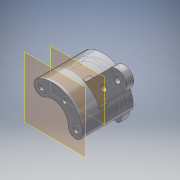
# Autodesk Inventor part: ChasssiPrototypeA2
Saved by Autodesk Inventor 2017 (Build 210142000, 142)
## iProperties
Created: 2018-04-20
Part Number: ChasssiPrototypeA2
Material: PC/ABS Plastic
Document SubType Name: Modeling
Designer: MtgSaber
Density: 0.357273 g/cm^3
Appearance: Smooth - White
Mass: 1.80108 g
Surface Area: 53.9114 cm^2
Volume: 5.04118 cm^3
Author: MtgSaber
Autodesk Inventor part; units mm, degrees
ref_plane "YZ Plane" through (0, 0, 0) normal (1, 0, 0) x (0, 1, 0)
ref_plane "XZ Plane" through (0, 0, 0) normal (0, 1, 0) x (-1, 0, 0)
ref_plane "Work Plane1" through (-76.8604, -25.4, 68.58) normal (0, 0, 1) x (0, -1, 0)
sketch "Sketch1" plane through (-76.8604, -25.4, 68.58) normal (0, 0, 1) x (0, -1, 0)
  circle A0 centre (-6.7107, -7.5406) radius 1.5875 construction
  circle A1 centre (-6.7107, 7.5406) radius 1.5875 construction
  circle A2 centre (6.35, 15.0812) radius 1.5875 construction
  circle A3 centre (19.4107, 7.5406) radius 1.5875 construction
  circle A4 centre (19.4107, -7.5406) radius 1.5875 construction
  circle A5 centre (6.35, -15.0813) radius 1.5875 construction
  circle A6 centre (15.0813, 0) radius 6.35 construction
  circle A7 centre (6.35, 0) radius 18.2562 construction
  arc A8 (6.35, 19.8437) -> (-10.8352, -9.9219) centre (6.35, 0) ccw
  arc A9 (-10.8352, -9.9219) -> (-2.5863, -5.1594) centre (-6.7107, -7.5406) ccw
  arc A10 (6.35, 10.3187) -> (6.35, 19.8437) centre (6.35, 15.0812) ccw
  arc A11 (6.35, 10.3187) -> (-2.5863, -5.1594) centre (6.35, 0) ccw
  point P0 (-25.4, 76.8604)
  dimension "d0" = 1.5875
  constraints: 8 point on circle, 4 centre point, 3 coincident, 3 tangent, 1 concentric
  measures "d0" radial gap between concentric circles of A7 A8
extrude "Extrusion1" add sketch "Sketch1" along normal blind 1.5875
sketch "Sketch2" plane through (-76.8604, -25.4, 70.1675) normal (0, 0, 1) x (1, 0, 0)
  circle A0 centre (-7.5406, 6.7107) radius 1.5875 projected
  circle A1 centre (7.5406, 6.7107) radius 1.5875 projected
  circle A2 centre (15.0812, -6.35) radius 1.5875 projected
  point P0 (76.8604, 25.4)
ref_plane "Work Plane2" through (-95.1167, -50.0063, 68.58) normal (0, 0, 1) x (1, 0, 0)
extrude "Extrusion2" cut sketch "Sketch2" against normal up to surface (1.5875 mm away)
sketch "Sketch3" plane through (-76.8604, -25.4, 68.58) normal (0, 0, -1) x (-1, 0, 0)
  circle A0 centre (0, -6.35) radius 18.2562 construction
  circle A1 centre (-7.5406, 6.7107) radius 1.5875 construction
  circle A2 centre (-15.0812, -6.35) radius 1.5875 construction
  circle A3 centre (7.5406, 6.7107) radius 1.5875 construction
  arc A4 (5.1594, 2.5863) -> (-10.3187, -6.35) centre (0, -6.35) ccw construction
  arc A5 (5.1594, 2.5863) -> (9.9219, 10.8352) centre (7.5406, 6.7107) ccw construction
  arc A6 (9.9219, 10.8352) -> (-19.8437, -6.35) centre (0, -6.35) ccw construction
  arc A7 (-19.8437, -6.35) -> (-10.3187, -6.35) centre (-15.0812, -6.35) ccw construction
  arc A8 (-19.8437, -6.35) -> (-10.3187, -6.35) centre (-15.0812, -6.35) ccw construction
  arc A9 (-19.8437, -6.35) -> (-17.8385, -10.2332) centre (-15.0812, -6.35) ccw
  arc A10 (9.9219, 10.8352) -> (-19.8437, -6.35) centre (0, -6.35) ccw
  arc A11 (5.1594, 2.5863) -> (9.9219, 10.8352) centre (7.5406, 6.7107) ccw construction
  arc A12 (12.2822, 7.157) -> (9.9219, 10.8352) centre (7.5406, 6.7107) ccw
  arc A13 (12.2822, 7.157) -> (-17.8385, -10.2332) centre (0, -6.35) ccw
  arc A14 (5.1594, 2.5863) -> (9.9219, 10.8352) centre (7.5406, 6.7107) ccw construction
  point P0 (-76.8604, 25.4)
  point P1 (-17.8385, -2.4668)
  point P2 (5.5563, 11.0402)
  constraints: 16 point on circle, 4 centre point, 4 coincident
extrude "Extrusion3" add sketch "Sketch3" along normal blind 31.75
sketch "Sketch4" plane through (-76.8604, -25.4, 36.83) normal (0, 0, -1) x (-1, 0, 0)
  circle A0 centre (0, -6.35) radius 15.875 construction
  arc A1 (12.2822, 7.157) -> (-17.8385, -10.2332) centre (0, -6.35) ccw construction
  line L0 (0, -6.35) -> (-7.9375, 7.3982) construction
  line L1 (-15.8104, -15.4781) -> (15.8104, 2.7781) construction
  arc A2 (-15.8104, -15.4781) -> (-12.4062, -16.2546) centre (-13.7482, -14.2875) ccw
  arc A3 (14.7808, -0.5582) -> (15.8104, 2.7781) centre (13.7482, 1.5875) ccw
  arc A4 (14.7808, -0.5582) -> (-12.4062, -16.2546) centre (0, -6.35) ccw
  arc A5 (15.8104, 2.7781) -> (-15.8104, -15.4781) centre (0, -6.35) ccw
  circle A6 centre (-7.5406, 6.7107) radius 1.5875 construction
  point P0 (-76.8604, 25.4)
  point P1 (-17.8385, -2.4668)
  point P2 (5.5563, 11.0402)
  constraints: 12 point on circle, 4 centre point, 4 end point, 3 coincident, 3 point on line, 2 concentric, 1 midpoint, 1 perpendicular
extrude "Extrusion4" add sketch "Sketch4" against normal blind 4.7625
ref_plane "Work Plane7" through (-76.8604, -25.4, 57.4675) normal (0, 0, 1) x (1, 0, 0)
sketch "Sketch7" plane through (-76.8604, -25.4, 57.4675) normal (0, 0, 1) x (1, 0, 0)
  arc A0 (19.8437, -6.35) -> (-9.9219, 10.8352) centre (0, -6.35) ccw construction
  arc A1 (17.8385, -10.2332) -> (-12.2822, 7.157) centre (0, -6.35) ccw construction
  line L0 (0, -6.35) -> (31.9505, 25.6005) construction
  line L1 (0, -6.35) -> (40.6249, -6.35) construction
  circle A2 centre (20.7668, 14.4168) radius 2.0574
  circle A3 centre (29.7471, 23.3971) radius 2.0574
  arc A4 (28.0319, 2.41) -> (2.9648, 22.8687) centre (0, -6.35) ccw construction
  arc A5 (34.2372, 18.907) -> (25.257, 27.8872) centre (29.7471, 23.3971) ccw
  line L2 (17.784, 2.4537) -> (34.2372, 18.907)
  line L3 (8.8037, 11.434) -> (25.257, 27.8872)
  arc A6 (17.784, 2.4537) -> (8.8037, 11.434) centre (0, -6.35) ccw
  point P0 (76.8604, 25.4)
  dimension "d22" = 45
  dimension "d24" = 4.1148
  dimension "d25" = 4.1148
  dimension "d26" = 12.7
  dimension "d27" = 9.525
  dimension "d29" = 12.7
  constraints: 8 end point, 8 point on circle, 5 centre point, 3 coincident, 2 point on line, 2 symmetric about line, 1 horizontal, 1 parallel, 1 tangent
  measures "d22" angle of L1 L0
  measures "d24" diameter of A2
  measures "d25" diameter of A3
  measures "d26" distance of A3.centre A2.centre
  measures "d27" radial gap between concentric circles of A0 A4
  measures "d29" diameter of A5
extrude "Extrusion6" add sketch "Sketch7" against normal blind 4.7625
fillet "Fillet1" radius 3.175 2 edges at (-68.0567, -13.966, 55.0862) (-59.0764, -22.9463, 55.0862)
body "Solid1"
